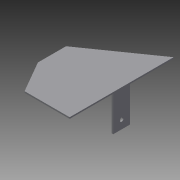
# Autodesk Inventor part: Left Chest
Saved by Autodesk Inventor 2014 (Build 180170000, 170)
## iProperties
Created: 2015-08-01
Part Number: Left Chest
Material: Generic
Document SubType Name: Modeling
Designer: Devon
Density: 1 g/cm^3
Appearance: Default
Author: Devon
Autodesk Inventor part; units mm, degrees
ref_plane "YZ Plane" through (0, 0, 0) normal (1, 0, 0) x (0, 1, 0)
ref_plane "XZ Plane" through (0, 0, 0) normal (0, 1, 0) x (-1, 0, 0)
ref_plane "XY Plane" through (0, 0, 0) normal (0, 0, 1) x (1, 0, 0)
sketch "Sketch1" plane through (0, 0, 0) normal (0, 1, 0) x (-1, 0, 0)
  line L0 (-24.4733, 28.5935) -> (-24.4733, -206.3565)
  line L1 (-24.4733, -206.3565) -> (118.5711, -106.1957)
  line L2 (-24.4733, -206.3565) -> (150.1517, -206.3565) construction
  line L3 (118.5711, -106.1957) -> (118.5711, -42.6957)
  line L4 (118.5711, -42.6957) -> (77.4122, 28.5935)
  line L5 (-24.4733, 28.5935) -> (77.4122, 28.5935)
  point P0 (0, 0)
  dimension "d0" = 234.95
  dimension "d1" = 174.625
  dimension "d2" = 35
  dimension "d3" = 63.5
  dimension "d4" = 150
  constraints: 12 end point, 2 perpendicular, 1 equal length, 1 horizontal, 1 vertical
  measures "d0" distance of L0.start L0.end
  measures "d1" distance of L0.end L1.end
  measures "d2" angle of L2 L1
  measures "d3" distance of L1.end L3.end
  measures "d4" angle of L4 L3
extrude "Extrusion1" add sketch "Sketch1" along normal blind 3.175
sketch "Sketch2" plane through (0, 0, 0) normal (0, -1, 0) x (1, 0, 0)
  line L0 (24.4733, 28.5935) -> (24.4733, -206.3565) projected
  line L1 (24.4733, 28.5935) -> (24.4733, -206.3565)
  line L2 (21.2983, -88.8815) -> (21.2983, -69.8315)
  line L3 (21.2983, -88.8815) -> (21.2983, -107.9315)
  line L4 (21.2983, -107.9315) -> (24.4733, -107.9315)
  line L5 (21.2983, -69.8315) -> (24.4733, -69.8315)
  point P0 (0, 0)
  dimension "d8" = 19.05
  dimension "d9" = 19.05
  constraints: 10 end point, 2 collinear, 2 perpendicular, 2 point on line, 1 parallel
  measures "d8" distance of L2.start L2.end
  measures "d9" distance of L2.start L3.end
extrude "Extrusion2" add sketch "Sketch2" along normal blind 79.2734
sketch "Sketch3" plane through (24.4733, 3.175, 28.5935) normal (1, 0, 0) x (0, 0, -1)
  line L0 (98.425, -82.4484) -> (117.475, -82.4484)
  line L1 (117.475, -82.4484) -> (117.475, -63.3984)
  line L2 (117.475, -63.3984) -> (98.425, -63.3984)
  line L3 (98.425, -63.3984) -> (98.425, -82.4484)
  point P0 (28.5935, -3.175)
  dimension "d12" = 19.05
  dimension "d13" = 19.05
  constraints: 8 end point, 2 parallel, 1 horizontal, 1 perpendicular
  measures "d12" distance of L2.end L1.end
  measures "d13" distance of L1.end L0.end
hole "Hole1" at (24.4733, -60.2234, -88.8815) direction (-1, 0, 0) diameter 8.3312 end through all
body "Solid1"
